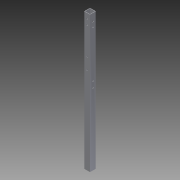
# Autodesk Inventor part: Edge Mount
Saved by Autodesk Inventor 2013 (Build 170138000, 138)
## iProperties
Created: 2013-01-21
Part Number: Edge Mount
Material: Aluminum 6061
Document SubType Name: Modeling
Designer: actoennies
Density: 2.71 g/cm^3
Mass: 242.128 g
Surface Area: 1134.04 cm^2
Volume: 89.3462 cm^3
Author: actoennies
Autodesk Inventor part; units mm, degrees
ref_plane "YZ Plane" through (0, 0, 0) normal (1, 0, 0) x (0, 1, 0)
ref_plane "XZ Plane" through (0, 0, 0) normal (0, 1, 0) x (-1, 0, 0)
ref_plane "XY Plane" through (0, 0, 0) normal (0, 0, 1) x (1, 0, 0)
sketch "Sketch1" plane through (0, 0, 0) normal (0, 1, 0) x (-1, 0, 0)
  line L0 (0, 0) -> (-25.4, 0)
  line L1 (-25.4, 0) -> (-25.4, 25.4)
  line L2 (-25.4, 25.4) -> (0, 25.4)
  line L3 (0, 25.4) -> (0, 0)
  line L4 (-1.5875, 23.8125) -> (-23.8125, 23.8125)
  line L5 (-23.8125, 23.8125) -> (-23.8125, 1.5875)
  line L6 (-23.8125, 1.5875) -> (-1.5875, 1.5875)
  line L7 (-1.5875, 1.5875) -> (-1.5875, 23.8125)
  dimension "d0" = 25.4
  dimension "d2" = 25.4
  dimension "d3" = 1.5875
  constraints: 16 end point, 4 parallel, 2 perpendicular, 1 horizontal, 3 other
  measures "d0" distance of L0.end L1.end
  measures "d2" distance of L1.end L2.end
  measures "d3" distance between parallel lines of L2 L4
extrude "Extrusion1" add sketch "Sketch1" along normal blind 596.9
sketch "Sketch7" plane through (25.4, 0, 0) normal (0, 0, -1) x (-1, 0, 0)
  circle A0 centre (12.7, 552.45) radius 3.3782
  circle A1 centre (12.7, 574.675) radius 3.3782
  constraints: 2 centre point, 4 other
extrude "Extrusion6" cut sketch "Sketch7" against normal blind 25.4
sketch "Sketch8" plane through (25.4, 0, 25.4) normal (1, 0, 0) x (0, 0, -1)
  circle A0 centre (12.7, 565.15) radius 3.3782
  circle A1 centre (12.7, 542.925) radius 3.3782
  constraints: 2 centre point, 4 other
extrude "Extrusion7" cut sketch "Sketch8" against normal blind 25.4
sketch "Sketch9" plane through (25.4, 0, 0) normal (0, 0, -1) x (-1, 0, 0)
  circle A0 centre (12.7, 431.8) radius 3.3782 projected
  line L0 (25.4, 440.055) -> (0, 440.055) projected
  line L1 (0, 368.3) -> (0, 440.055) projected
  line L2 (25.4, 368.3) -> (0, 368.3) projected
  line L3 (25.4, 440.055) -> (25.4, 368.3) projected
  circle A1 centre (12.7, 431.8) radius 3.3782 projected
  circle A2 centre (12.7, 381) radius 3.3782 projected
extrude "Extrusion8" cut sketch "Sketch9" against normal blind 25.4 contours A0 | A2
sketch "Sketch10" plane through (25.4, 0, 25.4) normal (1, 0, 0) x (0, 0, -1)
  circle A0 centre (12.7, 339.4075) radius 3.3782
  circle A1 centre (12.7, 314.0075) radius 3.3782
  constraints: 2 centre point, 4 other
extrude "Extrusion9" cut sketch "Sketch10" against normal blind 38.1
body "Solid1"
